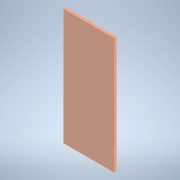
# Autodesk Inventor part: Door
Saved by Autodesk Inventor 2021 (Build 250183000, 183)
## iProperties
Created: 2021-07-31
Part Number: Door
Material: Wood (Oak)
Document SubType Name: Modeling
Designer: Shammy Haider
Density: 0.76 g/cm^3
Appearance: White Oak - Natural Medium Gloss
Author: Shammy Haider
Autodesk Inventor part; units mm, degrees
ref_plane "YZ Plane" through (0, 0, 0) normal (1, 0, 0) x (0, 1, 0)
ref_plane "XZ Plane" through (0, 0, 0) normal (0, 1, 0) x (-1, 0, 0)
ref_plane "XY Plane" through (0, 0, 0) normal (0, 0, 1) x (1, 0, 0)
sketch "Sketch1" plane through (0, 0, 0) normal (0, 0, 1) x (1, 0, 0)
  line L0 (460, -1050) -> (-460, -1050)
  line L1 (-460, -1050) -> (-460, 1050)
  line L2 (-460, 1050) -> (460, 1050)
  line L3 (460, 1050) -> (460, -1050)
  line L4 (460, -1050) -> (-460, 1050) construction
  line L5 (-460, -1050) -> (460, 1050) construction
  point P0 (0, 0)
  dimension "d0" = 2100
  dimension "d1" = 920
  constraints: 12 end point, 2 midpoint, 2 parallel, 1 horizontal, 1 perpendicular
  measures "d0" distance of L0.end L1.end
  measures "d1" distance of L0.start L0.end
extrude "Extrusion1" add sketch "Sketch1" along normal mid plane 40
sketch "Sketch2" plane through (460, -1050, 20) normal (1, 0, 0) x (0, 0, -1)
  line L0 (40, 1650) -> (0, 1650)
  line L1 (0, 1650) -> (0, 1750)
  line L2 (0, 1750) -> (40, 1750)
  line L3 (40, 1750) -> (40, 1650)
  line L4 (40, 1650) -> (0, 1750) construction
  line L5 (0, 1650) -> (40, 1750) construction
  line L6 (40, 2100) -> (40, 0) projected
  line L7 (0, 2100) -> (40, 2100) projected
  line L8 (40, 950) -> (0, 950)
  line L9 (0, 950) -> (0, 1050)
  line L10 (40, 1050) -> (40, 950)
  line L11 (0, 1050) -> (40, 1050)
  line L12 (40, 250) -> (0, 250)
  line L13 (0, 250) -> (0, 350)
  line L14 (40, 350) -> (40, 250)
  line L15 (0, 350) -> (40, 350)
  point P0 (20, 1050)
  point P1 (20, 1700)
  point P2 (40, 250)
  point P3 (40, 350)
  point P4 (40, 950)
  point P5 (40, 1050)
  dimension "d4" = 100
  dimension "d5" = 40
  dimension "d9" = 700
  dimension "d21" = 350
  constraints: 28 end point, 2 midpoint, 2 parallel, 1 collinear, 1 horizontal, 1 perpendicular, 1 vertical, 16 other
  measures "d4" distance of L2.end L0.start
  measures "d5" distance of L0.start L0.end
  measures "d9" distance of L0.start L8.start
  measures "d21" distance between parallel lines of L7 L2
extrude "Extrusion2" cut sketch "Sketch2" against normal blind 2.5
sketch "Sketch3" plane through (457.5, -1050, 20) normal (1, 0, 0) x (0, 0, -1)
  circle A0 centre (20, 1040) radius 4
  line L0 (0, 1050) -> (40, 1050) projected
  line L1 (40, 1050) -> (40, 950) projected
  point P0 (20, 1050)
  dimension "d16" = 8
  dimension "d17" = 10
  dimension "d18" = 20
  constraints: 1 centre point
  measures "d16" diameter of A0
  measures "d17" distance from line of L0 A0.centre
  measures "d18" distance from line of L1 A0.centre
extrude "Extrusion3" cut sketch "Sketch3" against normal blind 5
pattern_linear "Rectangular Pattern1" count 2 spacing 700 along (0, 1, 0) count 2 spacing 700 along (0, -1, 0) of "Extrusion3"
body "Solid1"
